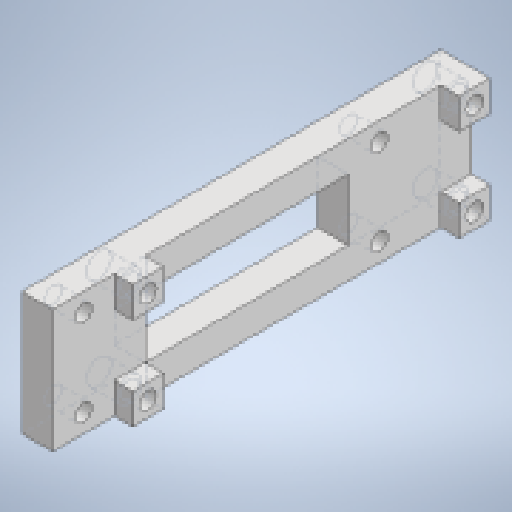
# Autodesk Inventor part: MotorDifferentialMountingBracket
Saved by Autodesk Inventor 2023 (Build 270158000, 158)
## iProperties
Created: 2023-03-28
Part Number: MotorDifferentialMountingBracket
Material: Generic
Document SubType Name: Modeling
Designer: Nathann
Density: 1 g/cm^3
Appearance: Default
Author: Nathann
Autodesk Inventor part; units mm, degrees
ref_plane "YZ Plane" through (0, 0, 0) normal (1, 0, 0) x (0, 1, 0)
ref_plane "XZ Plane" through (0, 0, 0) normal (0, 1, 0) x (-1, 0, 0)
ref_plane "XY Plane" through (0, 0, 0) normal (0, 0, 1) x (1, 0, 0)
sketch "Sketch1" plane through (0, 0, 0) normal (0, 1, 0) x (-1, 0, 0)
  line L0 (0, 0) -> (-5, 0)
  line L1 (-5, 0) -> (-5, 58)
  line L2 (-5, 58) -> (0, 58)
  line L3 (0, 58) -> (0, 0)
  line L4 (-5, 58) -> (-20, 58)
  line L5 (-20, 58) -> (-20, 53)
  line L6 (-20, 53) -> (-5, 53)
  line L7 (-5, 53) -> (-5, 58)
  line L8 (-5, 0) -> (-20, 0)
  line L9 (-20, 0) -> (-20, 5)
  line L10 (-20, 5) -> (-5, 5)
  line L11 (-5, 5) -> (-5, 0)
  point P0 (-5, 5)
  dimension "d0" = 5
  dimension "d1" = 5
  dimension "d2" = 5
  dimension "d3" = 15
  dimension "d4" = 15
  dimension "d5" = 48
  constraints: 24 end point, 6 parallel, 3 horizontal, 3 perpendicular, 1 point on line
  measures "d0" distance between parallel lines of L3 L1
  measures "d1" distance between parallel lines of L6 L4
  measures "d2" distance between parallel lines of L8 L10
  measures "d3" distance between parallel lines of L5 L1
  measures "d4" distance between parallel lines of L1 L9
  measures "d5" distance between parallel lines of L10 L6
extrude "Extrusion1" add sketch "Sketch1" along normal blind 20
sketch "Sketch2" plane through (0, 0, 58) normal (0, 0, 1) x (1, 0, 0)
  circle A0 centre (10, 10) radius 2.5
  line L0 (20, 0) -> (20, 20) projected
  line L1 (20, 0) -> (10, 0)
  line L2 (10, 0) -> (10, 20)
  line L3 (10, 20) -> (20, 20)
  line L4 (20, 20) -> (20, 0)
  line L5 (0, 0) -> (20, 0) projected
  line L6 (10, 4) -> (7, 4)
  line L7 (7, 4) -> (7, 16)
  line L8 (7, 16) -> (10, 16)
  line L9 (10, 16) -> (10, 4)
  dimension "d8" = 10
  dimension "d9" = 10
  dimension "d10" = 10
  dimension "d11" = 5
  dimension "d54" = 12
  dimension "d55" = 4
  dimension "d56" = 3
  constraints: 16 end point, 4 parallel, 2 horizontal, 2 perpendicular, 1 centre point, 1 point on line
  measures "d8" distance between parallel lines of L0 L2
  measures "d9" distance from line of L0 A0.centre
  measures "d10" distance from line of L5 A0.centre
  measures "d11" diameter of A0
  measures "d54" distance between parallel lines of L6 L8
  measures "d55" distance between parallel lines of L5 L6
  measures "d56" distance between parallel lines of L7 L2
extrude "Extrusion2" cut sketch "Sketch2" against normal blind 200 contours A0 L2 | A0 L2 L3 L0 L1 | L2 A0
sketch "Sketch3" plane through (0, 0, 0) normal (-1, 0, 0) x (0, 0, 1)
  line L0 (5, 0) -> (5, 20) projected
  line L1 (53, 0) -> (53, 20) projected
  line L2 (5, 15) -> (53, 15)
  line L3 (53, 15) -> (53, 5)
  line L4 (53, 5) -> (5, 5)
  line L5 (5, 5) -> (5, 15)
  line L6 (0, 20) -> (58, 20) projected
  line L7 (0, 0) -> (58, 0) projected
  point P0 (5, 5)
  dimension "d14" = 5
  dimension "d15" = 5
  constraints: 8 end point, 2 parallel, 2 point on line, 1 horizontal, 1 perpendicular
  measures "d14" distance between parallel lines of L6 L2
  measures "d15" distance between parallel lines of L7 L4
extrude "Extrusion3" cut sketch "Sketch3" against normal blind 20 contours L0 L2 L1 L4
sketch "Sketch4" plane through (0, 0, 0) normal (-1, 0, 0) x (0, 0, 1)
  line L0 (58, 0) -> (58, 20) projected
  line L1 (58, 20) -> (68, 20)
  line L2 (68, 20) -> (68, 0)
  line L3 (68, 0) -> (58, 0)
  line L4 (58, 0) -> (58, 20)
  line L5 (20, 20) -> (10.5196, 12.6519)
  line L6 (20, 20) -> (10, 20)
  line L7 (10, 20) -> (10, 0)
  line L8 (10, 0) -> (20, 0)
  line L9 (20, 0) -> (20, 20)
  circle A0 centre (63, 3) radius 1.375
  circle A1 centre (63, 17) radius 1.375
  circle A2 centre (15, 17) radius 1.375
  circle A3 centre (15, 3) radius 1.375
  line L10 (0, 0) -> (58, 0) projected
  line L11 (0, 20) -> (58, 20) projected
  line L12 (0, 0) -> (0, 20) projected
  point P0 (10.5196, 0.1519)
  point P1 (63, 20)
  dimension "d18" = 10
  dimension "d19" = 10
  dimension "d20" = 3
  dimension "d21" = 3
  dimension "d22" = 5
  dimension "d23" = 5
  dimension "d24" = 5
  dimension "d25" = 5
  dimension "d26" = 3
  dimension "d27" = 3
  dimension "d28" = 2.75
  dimension "d29" = 2.75
  dimension "d30" = 2.75
  dimension "d31" = 2.75
  dimension "d63" = 0
  dimension "d64" = 0
  dimension "d65" = 10
  constraints: 18 end point, 4 centre point, 4 parallel, 2 horizontal, 2 perpendicular, 1 midpoint, 1 point on line
  measures "d18" distance between parallel lines of L0 L2
  measures "d19" distance between parallel lines of L7 L9
  measures "d20" distance from line of L3 A0.centre
  measures "d21" distance of point (63, 20) A1.centre
  measures "d22" distance from line of L2 A0.centre
  measures "d23" distance from line of L2 A1.centre
  measures "d24" distance from line of L7 A2.centre
  measures "d25" distance from line of L7 A3.centre
  measures "d26" distance from line of L8 A3.centre
  measures "d27" distance from line of L6 A2.centre
  measures "d28" diameter of A0
  measures "d29" diameter of A1
  measures "d30" diameter of A2
  measures "d31" diameter of A3
  measures "d63" distance between parallel lines of L10 L8
  measures "d64" distance between parallel lines of L11 L6
  measures "d65" distance between parallel lines of L12 L7
extrude "Extrusion4" add sketch "Sketch4" against normal blind 5 contours L0 L1 L2 L3 | L8 L7 L6 L9
sketch "Sketch5" plane through (10, 12.5, 58) normal (1, 0, 0) x (0, 0, -1)
  circle A0 centre (55.5, 5) radius 1.375
  circle A1 centre (55.5, -10) radius 1.375
  circle A2 centre (2.5, 5) radius 1.375
  circle A3 centre (2.5, -10) radius 1.375
  line L0 (53, 7.5) -> (58, 7.5) projected
  line L1 (58, 7.5) -> (58, 0) projected
  line L2 (58, -5) -> (58, -12.5) projected
  line L3 (58, -12.5) -> (53, -12.5) projected
  line L4 (5, -12.5) -> (0, -12.5) projected
  line L5 (0, -12.5) -> (0, -5) projected
  line L6 (0, 0) -> (0, 7.5) projected
  line L7 (0, 7.5) -> (5, 7.5) projected
  dimension "d34" = 2.5
  dimension "d35" = 2.5
  dimension "d36" = 2.5
  dimension "d37" = 2.5
  dimension "d38" = 2.5
  dimension "d39" = 2.5
  dimension "d40" = 2.5
  dimension "d41" = 2.5
  dimension "d42" = 2.75
  dimension "d43" = 2.75
  dimension "d44" = 2.75
  dimension "d45" = 2.75
  constraints: 4 centre point
  measures "d34" distance from line of L0 A0.centre
  measures "d35" distance from line of L1 A0.centre
  measures "d36" distance from line of L2 A1.centre
  measures "d37" distance from line of L3 A1.centre
  measures "d38" distance from line of L4 A3.centre
  measures "d39" distance from line of L5 A3.centre
  measures "d40" distance from line of L6 A2.centre
  measures "d41" distance from line of L7 A2.centre
  measures "d42" diameter of A2
  measures "d43" diameter of A3
  measures "d44" diameter of A0
  measures "d45" diameter of A1
extrude "Extrusion5" cut sketch "Sketch5" against normal blind 15
sketch "Sketch6" plane through (0, 0, 68) normal (-1, 0, 0) x (0, 0, 1)
  circle A0 centre (-12.5, 17.5) radius 1.375 projected
  circle A1 centre (-12.5, 17.5) radius 2
  circle A2 centre (-12.5, 2.5) radius 1.375 projected
  circle A3 centre (-12.5, 2.5) radius 2
  circle A4 centre (-65.5, 2.5) radius 1.375 projected
  circle A5 centre (-65.5, 2.5) radius 2
  circle A6 centre (-65.5, 17.5) radius 1.375 projected
  circle A7 centre (-65.5, 17.5) radius 2
  point P0 (-68, 0)
  dimension "d48" = 4
  dimension "d49" = 4
  dimension "d50" = 4
  dimension "d51" = 4
  constraints: 4 centre point, 4 coincident
  measures "d48" diameter of A1
  measures "d49" diameter of A3
  measures "d50" diameter of A5
  measures "d51" diameter of A7
extrude "Extrusion6" cut sketch "Sketch6" against normal blind 3 contours A0 | A1 | A2 | A3 | A4 | A5 | A6 | A7
sketch "Sketch7" plane through (10, 10, 58) normal (0, 0, 1) x (1, 0, 0)
  line L0 (-10, -10) -> (-5, -10) projected
  line L1 (-5, -10) -> (-2, -10)
  line L2 (-2, -10) -> (-2, -5)
  line L3 (-2, -5) -> (-5, -5)
  line L4 (-5, -5) -> (-5, -10)
  line L5 (-5, 5) -> (-5, 10) projected
  line L6 (-5, 10) -> (-2, 10)
  line L7 (-2, 10) -> (-2, 5)
  line L8 (-2, 5) -> (-5, 5)
  line L9 (-5, 5) -> (-5, 10)
  line L10 (-5, 10) -> (-5, -10) projected
  line L11 (-5, -10) -> (0, -10) projected
  line L12 (0, -10) -> (0, -2.5) projected
  arc A0 (0, 2.5) -> (0, -2.5) centre (0, 0) ccw projected
  line L13 (0, 2.5) -> (0, 10) projected
  line L14 (-5, 10) -> (0, 10) projected
  point P0 (-2, 10)
  point P1 (-2, -10)
  dimension "d57" = 5
  dimension "d58" = 5
  dimension "d59" = 3
  dimension "d60" = 3
  constraints: 16 end point, 4 parallel, 2 horizontal, 2 perpendicular
  measures "d57" distance of L6.end L7.end
  measures "d58" distance of L1.end L2.end
  measures "d59" distance of L2.end L3.end
  measures "d60" distance of L7.end L8.end
extrude "Extrusion7" cut sketch "Sketch7" against normal blind 1000 contours L2 L3 L10 L8 L7 L14 L13 A0 L12 L11
sketch "Sketch8" plane through (0, 0, 0) normal (-1, 0, 0) x (0, 0, 1)
  circle A0 centre (2.5, 17.5) radius 2 projected
  circle A1 centre (55.5, 17.5) radius 2 projected
  circle A2 centre (2.5, 2.5) radius 2 projected
  circle A3 centre (55.5, 2.5) radius 2 projected
  line L0 (10, 5) -> (5, 5) projected
  line L1 (5, 5) -> (5, 15) projected
  line L2 (5, 15) -> (10, 15) projected
  line L3 (10, 15) -> (10, 5) projected
  circle A4 centre (63, 17) radius 1.375 projected
  circle A5 centre (63, 3) radius 1.375 projected
  line L4 (0, 0) -> (68, 0) projected
  line L5 (68, 0) -> (68, 20) projected
  line L6 (0, 20) -> (68, 20) projected
  line L7 (0, 0) -> (0, 20) projected
  line L8 (20, 5) -> (20, 15) projected
  line L9 (20, 15) -> (53, 15) projected
  line L10 (53, 15) -> (53, 5) projected
  line L11 (53, 5) -> (20, 5) projected
extrude "Extrusion8" add sketch "Sketch8" against normal blind 5 contours L0 L1 L2 L3
sketch "Sketch9" plane through (0, 0, 0) normal (-1, 0, 0) x (0, 0, 1)
  circle A0 centre (15, 17) radius 1.375
  circle A1 centre (15, 3) radius 1.375
  line L0 (68, 0) -> (68, 20) projected
  circle A2 centre (63, 3) radius 1.375 projected
  line L1 (0, 0) -> (68, 0) projected
  line L2 (0, 20) -> (68, 20) projected
  line L3 (20, 5) -> (20, 15) projected
  dimension "d68" = 5
  dimension "d69" = 3
  dimension "d70" = 3
  dimension "d71" = 3
  dimension "d72" = 5
  dimension "d73" = 5
  dimension "d74" = 2.75
  dimension "d75" = 2.75
  dimension "d76" = 2.75
  constraints: 2 centre point
  measures "d68" distance from line of L0 A2.centre
  measures "d69" distance from line of L1 A2.centre
  measures "d70" distance from line of L1 A1.centre
  measures "d71" distance from line of L2 A0.centre
  measures "d72" distance from line of L3 A0.centre
  measures "d73" distance from line of L3 A1.centre
  measures "d74" diameter of A2
  measures "d75" diameter of A1
  measures "d76" diameter of A0
extrude "Extrusion9" cut sketch "Sketch9" against normal blind 5 contours A0 | A1
sketch "Sketch10" plane through (0, 0, 0) normal (-1, 0, 0) x (0, 0, 1)
  line L0 (53, 5) -> (20, 5) projected
  line L1 (20, 5) -> (15, 5)
  line L2 (15, 5) -> (15, 15)
  line L3 (15, 15) -> (20, 15)
  line L4 (20, 15) -> (20, 5)
  point P0 (0, 0)
  dimension "d79" = 5
  constraints: 8 end point, 2 parallel, 1 horizontal, 1 perpendicular
  measures "d79" distance between parallel lines of L2 L4
extrude "Extrusion10" cut sketch "Sketch10" against normal blind 5
sketch "Sketch11" plane through (5, 0, 0) normal (1, 0, 0) x (0, 0, -1)
  circle A0 centre (-63, 17) radius 1.375 projected
  circle A1 centre (-63, 17) radius 2
  circle A2 centre (-63, 3) radius 1.375 projected
  circle A3 centre (-63, 3) radius 2
  circle A4 centre (-15, 3) radius 1.375 projected
  circle A5 centre (-15, 3) radius 2
  circle A6 centre (-15, 17) radius 1.375 projected
  circle A7 centre (-15, 17) radius 2
  point P0 (0, 0)
  dimension "d82" = 4
  dimension "d83" = 4
  dimension "d84" = 4
  dimension "d85" = 4
  constraints: 4 centre point, 4 coincident
  measures "d82" diameter of A1
  measures "d83" diameter of A3
  measures "d84" diameter of A5
  measures "d85" diameter of A7
extrude "Extrusion11" cut sketch "Sketch11" against normal blind 2 contours A0 | A1 | A2 | A3 | A4 | A5 | A6 | A7
equation "\"d14\" = d15"
equation "\"d19\" = d18"
equation "\"d20\" = d21"
equation "\"d24\" = d23"
equation "\"d25\" = d22"
equation "\"d26\" = d20"
equation "\"d27\" = d21"
equation "\"d34\" = d35"
equation "\"d37\" = d34"
equation "\"d38\" = d34"
equation "\"d39\" = d36"
equation "\"d40\" = d39"
equation "\"d41\" = d34"
equation "\"d44\" = d42"
equation "\"d45\" = d43"
equation "\"d49\" = d48"
equation "\"d50\" = d49"
equation "\"d51\" = d48"
equation "\"d75\" = d74"
equation "\"d76\" = d75"
body "Solid1"
